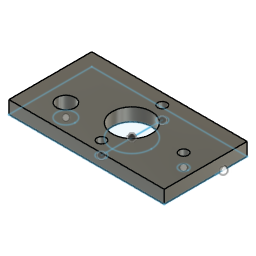
NoServoBraket (Autodesk Fusion 360 design; units mm, degrees)
Autodesk Fusion 360 part; units mm, degrees
sketch "Sketch1" plane through (0, 0, 0) normal (0, 0, 1) x (1, 0, 0)
  line L0 (20.1643, 5) -> (80.1643, 5)
  line L1 (80.1643, 5) -> (80.1643, 37)
  line L2 (80.1643, 37) -> (20.1643, 37)
  line L3 (20.1643, 37) -> (20.1643, 5)
  circle A0 centre (51.6483, 32.7576) radius 1.75
  circle A1 centre (51.6483, 9.2576) radius 1.75
  line L4 (51.6483, 32.7576) -> (51.6483, 9.2576)
  circle A2 centre (71.6483, 21.0076) radius 1.75
  circle A3 centre (32.1643, 15) radius 3.5
  line L5 (80.1643, 27.7253) -> (80.1643, 24.8327)
  circle A4 centre (51.6483, 21.0076) radius 7.5213
  dimension "d1" = 60
  dimension "d2" = 32
  dimension "d6" = 3.5
  dimension "d7" = 23.5
  dimension "d8" = 3.5
  dimension "d11" = 3.5
  dimension "d16" = 7
  dimension "d22" = 12
  dimension "d23" = 22
  dimension "d24" = 20
  dimension "d25" = 11.75
  constraint horizontal L0
  constraint vertical L1
  constraint horizontal L2
  constraint vertical L3
  constraint coincident A0.centre L4.start
  constraint coincident A1.centre L4.end
  constraint parallel L1 L4
  constraint vertical L5
  constraint coincident L1 L5.end
  constraint midpoint L4 A4.centre
  measures "d1" distance of L1.end L2.end
  measures "d2" distance of L0.start L2.end
  measures "d6" diameter of A0
  measures "d7" distance of A0.centre A1.centre
  measures "d8" diameter of A1
  measures "d11" diameter of A2
  measures "d16" diameter of A3
  measures "d22" distance of L3 A3.centre
  measures "d23" distance of L2 A3.centre
  measures "d24" distance of L4 A2.centre
  measures "d25" vertical distance of A1.centre A2.centre
extrude "Extrude5" add sketch "Sketch1" along normal blind 5
